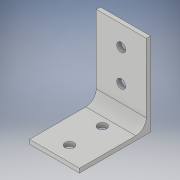
# Autodesk Inventor part: Triangle connector 2
Saved by Autodesk Inventor 2019 (Build 230136000, 136)
## iProperties
Created: 2020-10-22
Part Number: Triangle connector 2
Material: Generic
Document SubType Name: Modeling
Designer: Delta
Density: 1 g/cm^3
Appearance: Default
Author: Delta
Autodesk Inventor part; units mm, degrees
ref_plane "YZ Plane" through (0, 0, 0) normal (1, 0, 0) x (0, 1, 0)
ref_plane "XZ Plane" through (0, 0, 0) normal (0, 1, 0) x (-1, 0, 0)
ref_plane "XY Plane" through (0, 0, 0) normal (0, 0, 1) x (1, 0, 0)
sketch "Sketch1" plane through (0, 0, 0) normal (0, 0, 1) x (1, 0, 0)
  line L0 (0, 0) -> (15.24, 0)
  line L1 (15.24, 0) -> (15.24, 25.4)
  line L2 (15.24, 25.4) -> (0, 25.4)
  line L3 (0, 25.4) -> (0, 0)
  dimension "d0" = 25.4
  dimension "d1" = 15.24
  constraints: 8 end point, 2 parallel, 1 horizontal, 1 perpendicular
  measures "d0" distance of L0.end L1.end
  measures "d1" distance of L1.end L2.end
extrude "Extrusion1" add sketch "Sketch1" along normal blind 1.27
sketch "Sketch2" plane through (0, 0, 1.27) normal (0, 0, 1) x (1, 0, 0)
  line L0 (15.24, 0) -> (15.24, 25.4) projected
  line L1 (0, 0) -> (15.24, 0)
  line L2 (15.24, 0) -> (15.24, 1.27)
  line L3 (15.24, 1.27) -> (0, 1.27)
  line L4 (0, 1.27) -> (0, 0)
  dimension "d4" = 1.27
  constraints: 8 end point, 2 parallel, 1 horizontal, 1 perpendicular, 1 point on line
  measures "d4" distance between parallel lines of L1 L3
extrude "Extrusion2" add sketch "Sketch2" along normal blind 20.32
sketch "Sketch3" plane through (0, 0, 1.27) normal (0, 0, 1) x (1, 0, 0)
  circle A0 centre (7.62, 19.2024) radius 1.3589
  circle A1 centre (7.62, 9.5758) radius 1.3589
  line L0 (15.24, 1.27) -> (15.24, 25.4) projected
  line L1 (0, 0) -> (15.24, 0) projected
  dimension "d7" = 2.7178
  dimension "d8" = 2.7178
  dimension "d10" = 7.62
  dimension "d11" = 9.6266
  dimension "d25" = 9.5758
  dimension "d28" = 7.62
  constraints: 2 centre point
  measures "d7" diameter of A0
  measures "d8" diameter of A1
  measures "d10" distance from line of L0 A1.centre
  measures "d11" distance of A1.centre A0.centre
  measures "d25" distance from line of L1 A1.centre
  measures "d28" distance from line of L0 A0.centre
extrude "Extrusion3" cut sketch "Sketch3" against normal blind 25.4
sketch "Sketch4" plane through (0, 1.27, 26.67) normal (0, 1, 0) x (1, 0, 0)
  circle A0 centre (7.62, 19.6342) radius 1.3589
  circle A1 centre (7.62, 9.6266) radius 1.3589
  line L0 (20.32, 1.27) -> (20.32, 25.4)
  line L1 (0, 0) -> (20.32, 0)
  line L2 (15.24, 25.4) -> (15.24, 5.08) projected
  dimension "d19" = 2.7178
  dimension "d15" = 2.7178
  dimension "d17" = 10.0076
  dimension "d26" = 7.62
  dimension "d27" = 7.62
  constraints: 4 end point, 2 centre point
  measures "d19" diameter of A0
  measures "d15" diameter of A1
  measures "d17" distance of A1.centre A0.centre
  measures "d26" distance from line of L2 A1.centre
  measures "d27" distance from line of L2 A0.centre
extrude "Extrusion4" cut sketch "Sketch4" against normal blind 25.4
fillet "Fillet1" radius 3.175 1 edges at (7.62, 1.27, 1.27)
body "Solid1"
